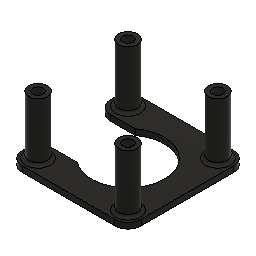
MotorMount_Low v5 (Autodesk Fusion 360 design; units mm, degrees)
Autodesk Fusion 360 part; units mm, degrees
sketch "Sketch1" plane through (0, 0, 0) normal (0, 1, 0) x (1, 0, 0)
  line L0 (0, 0) -> (41, 0)
  line L1 (41, 0) -> (41, -41)
  line L2 (41, -41) -> (0, -41)
  line L3 (0, -41) -> (0, 0)
  line L4 (0, -20.5) -> (41, -20.5) construction
  line L5 (20.5, 0) -> (20.5, -41) construction
  circle A0 centre (20.5, -20.5) radius 12.5
  line L6 (36, -36) -> (5, -36) construction
  line L7 (5, -36) -> (5, -5) construction
  line L8 (5, -5) -> (36, -5) construction
  line L9 (36, -5) -> (36, -36) construction
  line L10 (36, -36) -> (5, -5) construction
  line L11 (5, -36) -> (36, -5) construction
  circle A1 centre (5, -36) radius 1.8
  circle A2 centre (36, -36) radius 1.8
  circle A3 centre (36, -5) radius 1.8
  circle A4 centre (5, -5) radius 1.8
  circle A5 centre (5, -36) radius 3.25
  circle A6 centre (36, -36) radius 3.25
  circle A7 centre (36, -5) radius 3.25
  circle A8 centre (5, -5) radius 3.25
  line L12 (0, -10.5) -> (13, -10.5)
  line L13 (13, -30.5) -> (0, -30.5)
  point P0 (20.5, -20.5)
  dimension "d1" = 31
  dimension "d2" = 31
  dimension "d3" = 25
  dimension "d4" = 3.6
  dimension "d5" = 3.6
  dimension "d6" = 3.6
  dimension "d7" = 3.6
  dimension "d8" = 6.5
  dimension "d9" = 6.5
  dimension "d10" = 6.5
  dimension "d11" = 6.5
  dimension "d12" = 41
  dimension "d13" = 10
  dimension "d14" = 10
  constraint horizontal L0
  constraint vertical L1
  constraint horizontal L2
  constraint vertical L3
  constraint coincident L0.start L3.end
  constraint midpoint L3 L4.start
  constraint midpoint L1 L4.end
  constraint midpoint L0 L5.start
  constraint midpoint L2 L5.end
  constraint midpoint L5 P0
  constraint perpendicular L6 L7
  constraint parallel L6 L8
  constraint parallel L7 L9
  constraint horizontal L6
  constraint coincident L10 P0
  constraint coincident L11 P0
  constraint coincident P0 A0.centre
  constraint coincident L6.end L7.start
  constraint coincident L6.start L9.end
  constraint coincident L8.end L9.start
  constraint coincident L7.end L8.start
  constraint concentric A1 A5
  constraint concentric A2 A6
  constraint concentric A3 A7
  constraint concentric A4 A8
  constraint equal L0 L1
  constraint coincident L3 L12.start
  constraint coincident A0 L12.end
  constraint perpendicular L3 L12
  constraint coincident A0 L13.start
  constraint coincident L3 L13.end
  constraint perpendicular L3 L13
  measures "d1" distance of L6.start L8.end
  measures "d2" distance of L7.end L8.end
  measures "d3" diameter of A0
  measures "d4" diameter of A4
  measures "d5" diameter of A3
  measures "d6" diameter of A2
  measures "d7" diameter of A1
  measures "d8" diameter of A8
  measures "d9" diameter of A7
  measures "d10" diameter of A6
  measures "d11" diameter of A5
  measures "d12" distance of L0.start L0.end
  measures "d13" distance of L4 L12
  measures "d14" distance of L4 L13
extrude "Extrude1" add sketch "Sketch1" along normal blind 2 contours L0 L1 L2 L3 A0 L12 L13 | A5 | A6 | A7 | A8
extrude "Extrude2" add sketch "Sketch1" along normal blind 22 contours A5 | A6 | A7 | A8
ref_plane "WorkPlane1" through (20.5, 1, 20.5) normal (0, 0, 1) x (1, 0, 0)
fillet "Fillet1" radius 1 4 edges at (32.9699, 2, 34.8247) (32.9699, 2, 3.8247) (1.9699, 2, 3.8247) (1.9699, 2, 34.8247)
fillet "Fillet2" radius 4.5 6 edges at (41, 1, 0) (41, 1, 41) (0, 1, 0) (0, 1, 41) (0, 1, 10.5) (0, 1, 30.5)
equation "d2 = d1"
equation "d5 = d4"
equation "d6 = d5"
equation "d7 = d4"
equation "d9 = d8"
equation "d10 = d8"
equation "d11 = d8"
equation "d14 = d13"
equation "Hoogte = 22 mm"
equation "d18 = Hoogte"
equation "d20 = ( -41 / 2 ) * 1 mm"
